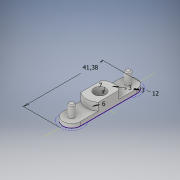
# Autodesk Inventor part: HarmonicDrive-WaveGenerator-Bottom
Saved by Autodesk Inventor 2018.3 (Build 223284000, 284)
## iProperties
Created: 2018-06-23
Part Number: HarmonicDrive-WaveGenerator-Bottom
Material: Generisch
Document SubType Name: Modeling
Designer: JochenAlt
Density: 1 g/cm^3
Appearance: Vorgabe
Author: JochenAlt
Autodesk Inventor part; units mm, degrees
ref_plane "YZ Plane" through (0, 0, 0) normal (1, 0, 0) x (0, 1, 0)
ref_plane "XZ Plane" through (0, 0, 0) normal (0, 1, 0) x (-1, 0, 0)
ref_plane "XY Plane" through (0, 0, 0) normal (0, 0, 1) x (1, 0, 0)
sketch "Skizze1" plane through (0, 0, 0) normal (0, 0, 1) x (1, 0, 0)
  line L0 (0, -14.6901) -> (0, 14.6901) construction
  line L1 (4.5, -14.6901) -> (4.5, 14.6901)
  line L2 (-4.5, 14.6901) -> (-4.5, -14.6901)
  arc A0 (-4.5, -14.6901) -> (4.5, -14.6901) centre (0, -14.6901) ccw
  arc A1 (4.5, 14.6901) -> (-4.5, 14.6901) centre (0, 14.6901) ccw
  line L3 (0, 28.9662) -> (0, -28.9662) construction
  line L4 (-8.4, 0) -> (8.4, 0) construction
  circle A2 centre (0, 14.6901) radius 1.5
  circle A3 centre (0, -14.6901) radius 1.5
  circle A4 centre (0, 0) radius 3
  circle A5 centre (0, 14.6901) radius 6 construction
  circle A6 centre (0, -14.6901) radius 6 construction
  line L5 (0, 20.6901) -> (0, -20.6901) construction
  arc A7 (-4.5, -5.3619) -> (4.5, -5.3619) centre (0, 0) ccw
  arc A8 (4.5, 5.3619) -> (-4.5, 5.3619) centre (0, 0) ccw
  dimension "d4" = 12
  dimension "d1" = 3
  dimension "d2" = 3
  dimension "d3" = 6
  dimension "d5" = 41.3803
  dimension "d13" = 7
  constraints: 10 end point, 8 point on circle, 7 centre point, 6 coincident, 6 point on line, 4 tangent, 2 equal radius, 2 vertical alignment, 1 midpoint, 1 parallel, 1 vertical, 5 other
  measures "d1" diameter of A2
  measures "d2" radial gap between concentric circles of A1 A2
  measures "d3" diameter of A4
  measures "d5" distance of L5.start L5.end
  measures "d13" radius of A8
extrude "Extrusion1" add sketch "Skizze1" along normal blind 2 contours A0 L2 A7 L1 | A7 L2 A8 L1 | A8 L2 A1 L1 | A2 | A3
extrude "Extrusion2" add sketch "Skizze1" along normal blind 8 contours A2 | A3
chamfer "Fase1" distance 0.5 angle 45 2 edges at (-1.5, -14.6901, 8) (-1.5, 14.6901, 8)
extrude "Extrusion3" add sketch "Skizze1" along normal blind 6 contours A7 L2 A8 L1
